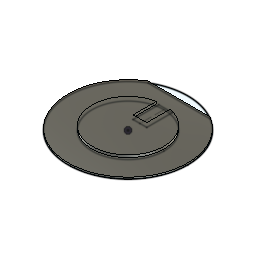
płytka_pop v2 (Autodesk Fusion 360 design; units mm, degrees)
Autodesk Fusion 360 part; units mm, degrees
sketch "Szkic1" plane through (0, 0, 0) normal (0, 0, 1) x (1, 0, 0)
  circle A0 centre (0, 0) radius 10.5
  line L0 (0, 10.5) -> (0, 3.5) construction
  line L1 (0, 3.5) -> (2, 3.5)
  line L2 (2, 3.5) -> (2, 11)
  line L3 (2, 11) -> (-2, 11)
  line L4 (-2, 11) -> (-2, 3.5)
  line L5 (-2, 3.5) -> (0, 3.5)
  circle A1 centre (0, 0) radius 17.5
  line L6 (9.089, 14.9546) -> (-9.089, 14.9546)
  dimension "d1" = 21
  dimension "d2" = 7
  dimension "d3" = 2
  dimension "d4" = 3.5
  dimension "d5" = 2
  dimension "d6" = 3.5
  dimension "d7" = 0.5
  dimension "d10" = 35
  dimension "d15" = 18.1779
  constraint coincident A0.centre A1.centre
  constraint coincident A0 L0.start
  constraint vertical L0
  constraint perpendicular L0 L1
  constraint perpendicular L1 L2
  constraint perpendicular L2 L3
  constraint perpendicular L1 L4
  constraint perpendicular L0 L5
  constraint coincident A1 L6.start
  constraint coincident A1 L6.end
  constraint horizontal L6
  measures "d1" diameter of A0
  measures "d2" distance of L0.start L0.end
  measures "d3" distance of L0.end L1.end
  measures "d4" distance of A0.centre L0.end
  measures "d5" distance of L0.end L4.end
  measures "d6" distance of A0.centre L1
  measures "d7" distance of L0.start L3
  measures "d10" diameter of A1
  measures "d15" distance of L6.start L6.end
extrude "Wyciągnięcie proste1" add sketch "Szkic1" along normal blind 1 contours A0 L1 L2 L4 L5 picked at (1.5608, -1.0505)
extrude "Wyciągnięcie proste2" add sketch "Szkic1" along normal blind 0.5 contours A0 L1 L2 L4 L5 | A0 L2 L3 L4 | A1 L6 picked at (-1.3333, 5.7693) picked at (0.6667, 13.6364)
extrude "Wyciągnięcie proste3" add 1 faces at (0, -1.1667, 1) along direction (0, 0, 1) blind 0.2
